Autodesk Fusion 360 part; units mm, degrees
(part 11 of 20)
  spline S1104 degree 3 poles (20.0046, -835.3457) (19.913, -835.5599) (19.6837, -836.0959) (19.6861, -836.6821) (19.6875, -837.034) knots 0 0 0 0 0.069271 0.173342 0.173342 0.173342 0.173342
sketch "Boceto14" plane through (0, -1, 0) normal (0, -1, 0) x (1, 0, 0)
  line L0 (28.545, -839.4996) -> (28.5449, -835.8775)
  line L1 (28.5449, -835.8775) -> (29.094, -835.8775)
  line L2 (29.094, -835.8775) -> (29.094, -836.3857)
  spline S0 degree 3 poles (29.094, -836.3857) (29.1559, -836.3011) (29.2808, -836.1306) (29.4582, -836.0156) (29.5476, -835.9576) knots 0 0 0 0 0.031158 0.062835 0.062835 0.062835 0.062835
  spline S1 degree 3 poles (29.5476, -835.9576) (29.6468, -835.9104) (29.8507, -835.8133) (30.0763, -835.8016) (30.1922, -835.7956) knots 0 0 0 0 0.032617 0.067048 0.067048 0.067048 0.067048
  spline S2 degree 3 poles (30.1922, -835.7956) (30.3167, -835.8003) (30.5491, -835.8092) (30.7561, -835.914) (30.8522, -835.9627) knots 0 0 0 0 0.036859 0.068796 0.068796 0.068796 0.068796
  spline S3 degree 3 poles (30.8522, -835.9627) (30.9319, -836.0244) (31.0928, -836.1491) (31.1743, -836.3357) (31.2154, -836.4299) knots 0 0 0 0 0.029725 0.060035 0.060035 0.060035 0.060035
  spline S4 degree 3 poles (31.2154, -836.4299) (31.3656, -836.245) (31.6567, -835.8864) (32.1131, -835.8252) (32.3341, -835.7955) knots 0 0 0 0 0.068625 0.133024 0.133024 0.133024 0.133024
  spline S5 degree 3 poles (32.3341, -835.7955) (32.4992, -835.8039) (32.8071, -835.8196) (33.0502, -836.007) (33.1629, -836.0939) knots 0 0 0 0 0.048244 0.08997 0.08997 0.08997 0.08997
  spline S6 degree 3 poles (33.1629, -836.0939) (33.2472, -836.2162) (33.4366, -836.4911) (33.4471, -836.8268) (33.4528, -837.0131) knots 0 0 0 0 0.043695 0.098195 0.098195 0.098195 0.098195
  line L3 (33.4528, -837.0131) -> (33.4529, -839.4994)
  line L4 (33.4529, -839.4994) -> (32.8424, -839.4995)
  line L5 (32.8424, -839.4995) -> (32.8423, -837.2177)
  spline S7 degree 3 poles (32.8423, -837.2177) (32.8423, -837.1115) (32.8423, -836.9322) (32.7999, -836.7583) (32.7826, -836.6874) knots 0 0 0 0 0.031711 0.053535 0.053535 0.053535 0.053535
  spline S8 degree 3 poles (32.7826, -836.6874) (32.7582, -836.6357) (32.7084, -836.5303) (32.6141, -836.4615) (32.5661, -836.4265) knots 0 0 0 0 0.016863 0.034394 0.034394 0.034394 0.034394
  spline S9 degree 3 poles (32.5661, -836.4265) (32.5103, -836.3976) (32.3949, -836.3379) (32.2649, -836.3311) (32.1977, -836.3276) knots 0 0 0 0 0.018597 0.038532 0.038532 0.038532 0.038532
  spline S10 degree 3 poles (32.1977, -836.3276) (32.0766, -836.3374) (31.8386, -836.3566) (31.654, -836.5076) (31.5633, -836.5817) knots 0 0 0 0 0.035532 0.069798 0.069798 0.069798 0.069798
  spline S11 degree 3 poles (31.5633, -836.5817) (31.49, -836.6884) (31.3229, -836.9316) (31.3153, -837.2285) (31.311, -837.3951) knots 0 0 0 0 0.038079 0.086792 0.086792 0.086792 0.086792
  line L6 (31.311, -837.3951) -> (31.311, -839.4995)
  line L7 (31.311, -839.4995) -> (30.6971, -839.4995)
  line L8 (30.6971, -839.4995) -> (30.697, -837.1462)
  spline S12 degree 3 poles (30.697, -837.1462) (30.6946, -837.0241) (30.6903, -836.8074) (30.5906, -836.6159) (30.547, -836.5323) knots 0 0 0 0 0.036008 0.063954 0.063954 0.063954 0.063954
  spline S13 degree 3 poles (30.547, -836.5323) (30.4847, -836.4727) (30.3485, -836.3423) (30.1589, -836.3328) (30.0558, -836.3277) knots 0 0 0 0 0.025037 0.054812 0.054812 0.054812 0.054812
  spline S14 degree 3 poles (30.0558, -836.3277) (29.9711, -836.3333) (29.8016, -836.3447) (29.6516, -836.4243) (29.5766, -836.4641) knots 0 0 0 0 0.025172 0.050327 0.050327 0.050327 0.050327
  spline S15 degree 3 poles (29.5766, -836.4641) (29.508, -836.5158) (29.3677, -836.6214) (29.2949, -836.7814) (29.2577, -836.8631) knots 0 0 0 0 0.025339 0.051812 0.051812 0.051812 0.051812
  spline S16 degree 3 poles (29.2577, -836.8631) (29.229, -836.9694) (29.1622, -837.217) (29.1601, -837.4738) (29.1589, -837.6203) knots 0 0 0 0 0.032907 0.076633 0.076633 0.076633 0.076633
  line L9 (29.1589, -837.6203) -> (29.1589, -839.4996)
  line L10 (29.1589, -839.4996) -> (28.545, -839.4996)
  line L11 (19.0617, -788.1561) -> (19.7063, -788.1015)
  spline S17 degree 3 poles (19.7063, -788.1015) (19.734, -788.2447) (19.7853, -788.5096) (19.9591, -788.7149) (20.0389, -788.8091) knots 0 0 0 0 0.042908 0.079365 0.079365 0.079365 0.079365
  spline S18 degree 3 poles (20.0389, -788.8091) (20.1311, -788.8783) (20.3177, -789.0182) (20.5504, -789.0368) (20.6682, -789.0461) knots 0 0 0 0 0.033826 0.068485 0.068485 0.068485 0.068485
  spline S19 degree 3 poles (20.6682, -789.0461) (20.8106, -789.0318) (21.0974, -789.003) (21.311, -788.8093) (21.4185, -788.7118) knots 0 0 0 0 0.041772 0.0841 0.0841 0.0841 0.0841
  spline S20 degree 3 poles (21.4185, -788.7118) (21.508, -788.5868) (21.6971, -788.3223) (21.7156, -787.9967) (21.7254, -787.825) knots 0 0 0 0 0.045186 0.095569 0.095569 0.095569 0.095569
  spline S21 degree 3 poles (21.7254, -787.825) (21.7163, -787.6627) (21.6992, -787.3564) (21.5163, -787.1114) (21.4303, -786.9963) knots 0 0 0 0 0.047557 0.089725 0.089725 0.089725 0.089725
  spline S22 degree 3 poles (21.4303, -786.9963) (21.3218, -786.9078) (21.0972, -786.7246) (20.8075, -786.7036) (20.6578, -786.6928) knots 0 0 0 0 0.040971 0.08482 0.08482 0.08482 0.08482
  spline S23 degree 3 poles (20.6578, -786.6928) (20.5622, -786.6979) (20.3748, -786.708) (20.2053, -786.7883) (20.1223, -786.8275) knots 0 0 0 0 0.028423 0.055689 0.055689 0.055689 0.055689
  spline S24 degree 3 poles (20.1223, -786.8275) (20.0475, -786.8751) (19.9006, -786.9683) (19.7977, -787.1085) (19.7472, -787.1772) knots 0 0 0 0 0.026342 0.051681 0.051681 0.051681 0.051681
  line L12 (19.7472, -787.1772) -> (19.1708, -787.1022)
  line L13 (19.1708, -787.1022) -> (19.6549, -784.5339)
  line L14 (19.6549, -784.5339) -> (22.1413, -784.5337)
  line L15 (22.1413, -784.5337) -> (22.1413, -785.1204)
  line L16 (22.1413, -785.1204) -> (20.1461, -785.1205)
  line L17 (20.1461, -785.1205) -> (19.8767, -786.4643)
  spline S25 degree 3 poles (19.8767, -786.4643) (20.0262, -786.3728) (20.3171, -786.1948) (20.6565, -786.165) (20.8215, -786.1505) knots 0 0 0 0 0.051785 0.100763 0.100763 0.100763 0.100763
  spline S26 degree 3 poles (20.8215, -786.1505) (21.0307, -786.1688) (21.4463, -786.2053) (21.7672, -786.4717) (21.9265, -786.604) knots 0 0 0 0 0.061424 0.122014 0.122014 0.122014 0.122014
  spline S27 degree 3 poles (21.9265, -786.604) (22.0578, -786.7694) (22.3287, -787.1108) (22.3605, -787.5461) (22.3768, -787.7704) knots 0 0 0 0 0.061868 0.127641 0.127641 0.127641 0.127641
  spline S28 degree 3 poles (22.3768, -787.7704) (22.3616, -787.9874) (22.3318, -788.4132) (22.0967, -788.7691) (21.9813, -788.9437) knots 0 0 0 0 0.064036 0.125703 0.125703 0.125703 0.125703
  spline S29 degree 3 poles (21.9813, -788.9437) (21.8036, -789.1208) (21.4405, -789.4825) (20.9292, -789.5278) (20.6682, -789.5509) knots 0 0 0 0 0.072854 0.148822 0.148822 0.148822 0.148822
  spline S30 degree 3 poles (20.6682, -789.5509) (20.455, -789.5382) (20.0475, -789.5138) (19.7138, -789.2803) (19.5546, -789.169) knots 0 0 0 0 0.062678 0.119794 0.119794 0.119794 0.119794
  spline S31 degree 3 poles (19.5546, -789.169) (19.426, -789.0286) (19.1617, -788.7403) (19.0956, -788.3542) (19.0617, -788.1561) knots 0 0 0 0 0.055877 0.114795 0.114795 0.114795 0.114795
  line L18 (27.4212, -788.1384) -> (28.0249, -788.2168)
  spline S32 degree 3 poles (28.0249, -788.2168) (27.9822, -788.4107) (27.9005, -788.7824) (27.6421, -789.0608) (27.5185, -789.194) knots 0 0 0 0 0.058356 0.111856 0.111856 0.111856 0.111856
  spline S33 degree 3 poles (27.5185, -789.194) (27.3724, -789.2969) (27.0723, -789.5084) (26.7057, -789.5339) (26.5175, -789.5471) knots 0 0 0 0 0.052559 0.107965 0.107965 0.107965 0.107965
  spline S34 degree 3 poles (26.5175, -789.5471) (26.2844, -789.5296) (25.8328, -789.4957) (25.4886, -789.2028) (25.322, -789.0611) knots 0 0 0 0 0.068154 0.132052 0.132052 0.132052 0.132052
  spline S35 degree 3 poles (25.322, -789.0611) (25.1905, -788.8704) (24.9026, -788.453) (24.8815, -787.9442) (24.87, -787.6679) knots 0 0 0 0 0.068157 0.149141 0.149141 0.149141 0.149141
  spline S36 degree 3 poles (24.87, -787.6679) (24.8763, -787.4827) (24.8883, -787.1302) (25.0077, -786.7986) (25.0643, -786.6413) knots 0 0 0 0 0.055211 0.105055 0.105055 0.105055 0.105055
  spline S37 degree 3 poles (25.0643, -786.6413) (25.1365, -786.5044) (25.2787, -786.2348) (25.5316, -786.0649) (25.656, -785.9813) knots 0 0 0 0 0.04564 0.089884 0.089884 0.089884 0.089884
  spline S38 degree 3 poles (25.656, -785.9813) (25.792, -785.9171) (26.0658, -785.7878) (26.3683, -785.7701) (26.5206, -785.7612) knots 0 0 0 0 0.044643 0.089955 0.089955 0.089955 0.089955
  spline S39 degree 3 poles (26.5206, -785.7612) (26.7043, -785.7706) (27.0522, -785.7884) (27.3468, -785.9726) (27.4858, -786.0596) knots 0 0 0 0 0.054149 0.102527 0.102527 0.102527 0.102527
  spline S40 degree 3 poles (27.4858, -786.0596) (27.6003, -786.1731) (27.8394, -786.4101) (27.9232, -786.7368) (27.9668, -786.9071) knots 0 0 0 0 0.047449 0.099081 0.099081 0.099081 0.099081
  line L19 (27.9668, -786.9071) -> (27.3699, -786.9992)
  spline S41 degree 3 poles (27.3699, -786.9992) (27.3391, -786.8878) (27.2816, -786.6804) (27.1356, -786.523) (27.0681, -786.4501) knots 0 0 0 0 0.034086 0.063475 0.063475 0.063475 0.063475
  spline S42 degree 3 poles (27.0681, -786.4501) (26.9911, -786.3964) (26.8338, -786.2867) (26.6423, -786.273) (26.5445, -786.266) knots 0 0 0 0 0.027619 0.056426 0.056426 0.056426 0.056426
  spline S43 degree 3 poles (26.5445, -786.266) (26.3979, -786.2791) (26.1087, -786.3048) (25.8958, -786.5016) (25.7908, -786.5986) knots 0 0 0 0 0.04285 0.084486 0.084486 0.084486 0.084486
  spline S44 degree 3 poles (25.7908, -786.5986) (25.7066, -786.7382) (25.5128, -787.0597) (25.5052, -787.4372) (25.501, -787.6508) knots 0 0 0 0 0.048123 0.11083 0.11083 0.11083 0.11083
  spline S45 degree 3 poles (25.501, -787.6508) (25.5046, -787.8666) (25.5109, -788.2453) (25.6995, -788.5712) (25.7807, -788.7115) knots 0 0 0 0 0.063398 0.111295 0.111295 0.111295 0.111295
  spline S46 degree 3 poles (25.7807, -788.7115) (25.8819, -788.808) (26.0864, -789.0031) (26.3682, -789.0291) (26.5106, -789.0423) knots 0 0 0 0 0.040675 0.082263 0.082263 0.082263 0.082263
  spline S47 degree 3 poles (26.5106, -789.0423) (26.625, -789.0341) (26.8478, -789.018) (27.0271, -788.8852) (27.1143, -788.8205) knots 0 0 0 0 0.033628 0.065508 0.065508 0.065508 0.065508
  spline S48 degree 3 poles (27.1143, -788.8205) (27.1883, -788.7306) (27.3518, -788.5319) (27.3967, -788.2775) (27.4212, -788.1384) knots 0 0 0 0 0.034396 0.07593 0.07593 0.07593 0.07593
  spline S49 degree 3 poles (21.7321, -737.034) (21.7357, -736.7657) (21.7422, -736.2825) (21.8615, -735.8147) (21.9145, -735.6066) knots 0 0 0 0 0.080152 0.144341 0.144341 0.144341 0.144341
  spline S50 degree 3 poles (21.9145, -735.6066) (21.9791, -735.4398) (22.1017, -735.1233) (22.3428, -734.8853) (22.4568, -734.7727) knots 0 0 0 0 0.052977 0.10048 0.10048 0.10048 0.10048
  spline S51 degree 3 poles (22.4568, -734.7727) (22.5882, -734.6872) (22.863, -734.5083) (23.1911, -734.4893) (23.3623, -734.4794) knots 0 0 0 0 0.046203 0.096661 0.096661 0.096661 0.096661
  spline S52 degree 3 poles (23.3623, -734.4794) (23.4901, -734.485) (23.7356, -734.4957) (23.9605, -734.5941) (24.0683, -734.6414) knots 0 0 0 0 0.037989 0.072993 0.072993 0.072993 0.072993
  spline S53 degree 3 poles (24.0683, -734.6414) (24.1655, -734.7021) (24.3629, -734.8252) (24.5001, -735.0132) (24.5697, -735.1086) knots 0 0 0 0 0.034048 0.069103 0.069103 0.069103 0.069103
  spline S54 degree 3 poles (24.5697, -735.1086) (24.633, -735.2196) (24.767, -735.4545) (24.841, -735.7148) (24.8801, -735.8521) knots 0 0 0 0 0.038176 0.080832 0.080832 0.080832 0.080832
  spline S55 degree 3 poles (24.8801, -735.8521) (24.9128, -736.0232) (24.9874, -736.4133) (24.9907, -736.8107) (24.9926, -737.0339) knots 0 0 0 0 0.052146 0.118926 0.118926 0.118926 0.118926
  spline S56 degree 3 poles (24.9926, -737.0339) (24.989, -737.3005) (24.9824, -737.7813) (24.8645, -738.247) (24.8119, -738.4544) knots 0 0 0 0 0.079639 0.143634 0.143634 0.143634 0.143634
  spline S57 degree 3 poles (24.8119, -738.4544) (24.7477, -738.6214) (24.6259, -738.9384) (24.3852, -739.1771) (24.2713, -739.2901) knots 0 0 0 0 0.052961 0.100531 0.100531 0.100531 0.100531
  spline S58 degree 3 poles (24.2713, -739.2901) (24.1397, -739.3761) (23.864, -739.5562) (23.5346, -739.5752) (23.3624, -739.5851) knots 0 0 0 0 0.046339 0.097057 0.097057 0.097057 0.097057
  spline S59 degree 3 poles (23.3624, -739.5851) (23.1362, -739.5658) (22.6949, -739.5281) (22.3801, -739.2179) (22.2267, -739.0667) knots 0 0 0 0 0.065835 0.128409 0.128409 0.128409 0.128409
  spline S60 degree 3 poles (22.2267, -739.0667) (22.0832, -738.7986) (21.7456, -738.1676) (21.737, -737.4479) (21.7321, -737.034) knots 0 0 0 0 0.090022 0.211899 0.211899 0.211899 0.211899
  line L20 (28.1509, -738.173) -> (28.7546, -738.2514)
  spline S61 degree 3 poles (28.7546, -738.2514) (28.7119, -738.4453) (28.6302, -738.8171) (28.3717, -739.0954) (28.2481, -739.2286) knots 0 0 0 0 0.058356 0.111856 0.111856 0.111856 0.111856
  spline S62 degree 3 poles (28.2481, -739.2286) (28.1021, -739.3315) (27.802, -739.543) (27.4353, -739.5685) (27.2471, -739.5816) knots 0 0 0 0 0.052559 0.107965 0.107965 0.107965 0.107965
  spline S63 degree 3 poles (27.2471, -739.5816) (27.0141, -739.5641) (26.5625, -739.5302) (26.2182, -739.2373) (26.0517, -739.0956) knots 0 0 0 0 0.068154 0.132052 0.132052 0.132052 0.132052
  spline S64 degree 3 poles (26.0517, -739.0956) (25.9201, -738.9049) (25.6323, -738.4875) (25.6112, -737.9787) (25.5997, -737.7024) knots 0 0 0 0 0.068157 0.149141 0.149141 0.149141 0.149141
  spline S65 degree 3 poles (25.5997, -737.7024) (25.6061, -737.5171) (25.6181, -737.1646) (25.7375, -736.8331) (25.7941, -736.6758) knots 0 0 0 0 0.055211 0.105055 0.105055 0.105055 0.105055
  spline S66 degree 3 poles (25.7941, -736.6758) (25.8663, -736.5389) (26.0085, -736.2693) (26.2614, -736.0994) (26.3859, -736.0158) knots 0 0 0 0 0.04564 0.089884 0.089884 0.089884 0.089884
  spline S67 degree 3 poles (26.3859, -736.0158) (26.5218, -735.9516) (26.7957, -735.8223) (27.0981, -735.8047) (27.2505, -735.7958) knots 0 0 0 0 0.044643 0.089956 0.089956 0.089956 0.089956
  spline S68 degree 3 poles (27.2505, -735.7958) (27.4342, -735.8052) (27.7821, -735.8229) (28.0767, -736.0072) (28.2157, -736.0942) knots 0 0 0 0 0.054149 0.102527 0.102527 0.102527 0.102527
  spline S69 degree 3 poles (28.2157, -736.0942) (28.3301, -736.2077) (28.5692, -736.4447) (28.6529, -736.7715) (28.6966, -736.9417) knots 0 0 0 0 0.047449 0.099081 0.099081 0.099081 0.099081
  line L21 (28.6966, -736.9417) -> (28.0997, -737.0338)
  spline S70 degree 3 poles (28.0997, -737.0338) (28.0689, -736.9224) (28.0114, -736.715) (27.8654, -736.5576) (27.7979, -736.4847) knots 0 0 0 0 0.034086 0.063475 0.063475 0.063475 0.063475
  spline S71 degree 3 poles (27.7979, -736.4847) (27.7209, -736.431) (27.5636, -736.3213) (27.3721, -736.3076) (27.2743, -736.3006) knots 0 0 0 0 0.027619 0.056426 0.056426 0.056426 0.056426
  spline S72 degree 3 poles (27.2743, -736.3006) (27.1277, -736.3136) (26.8385, -736.3393) (26.6256, -736.5361) (26.5206, -736.6331) knots 0 0 0 0 0.04285 0.084486 0.084486 0.084486 0.084486
  spline S73 degree 3 poles (26.5206, -736.6331) (26.4364, -736.7727) (26.2425, -737.0942) (26.235, -737.4717) (26.2307, -737.6853) knots 0 0 0 0 0.048123 0.11083 0.11083 0.11083 0.11083
  spline S74 degree 3 poles (26.2307, -737.6853) (26.2343, -737.9011) (26.2406, -738.2798) (26.4292, -738.6057) (26.5104, -738.746) knots 0 0 0 0 0.063398 0.111295 0.111295 0.111295 0.111295
  spline S75 degree 3 poles (26.5104, -738.746) (26.6116, -738.8425) (26.8161, -739.0376) (27.0979, -739.0637) (27.2403, -739.0768) knots 0 0 0 0 0.040675 0.082263 0.082263 0.082263 0.082263
  spline S76 degree 3 poles (27.2403, -739.0768) (27.3547, -739.0686) (27.5775, -739.0526) (27.7568, -738.9198) (27.844, -738.8551) knots 0 0 0 0 0.033628 0.065508 0.065508 0.065508 0.065508
  spline S77 degree 3 poles (27.844, -738.8551) (27.918, -738.7651) (28.0815, -738.5665) (28.1264, -738.3121) (28.1509, -738.173) knots 0 0 0 0 0.034396 0.07593 0.07593 0.07593 0.07593
  line L22 (21.7306, -688.1902) -> (22.3752, -688.1357)
  spline S78 degree 3 poles (22.3752, -688.1357) (22.4029, -688.2789) (22.4541, -688.5438) (22.6279, -688.7491) (22.7077, -688.8434) knots 0 0 0 0 0.042908 0.079365 0.079365 0.079365 0.079365
  spline S79 degree 3 poles (22.7077, -688.8434) (22.7999, -688.9125) (22.9865, -689.0525) (23.2192, -689.071) (23.337, -689.0804) knots 0 0 0 0 0.033826 0.068485 0.068485 0.068485 0.068485
  spline S80 degree 3 poles (23.337, -689.0804) (23.4794, -689.0661) (23.7662, -689.0373) (23.9798, -688.8436) (24.0873, -688.7462) knots 0 0 0 0 0.041772 0.0841 0.0841 0.0841 0.0841
  spline S81 degree 3 poles (24.0873, -688.7462) (24.1768, -688.6211) (24.366, -688.3566) (24.3845, -688.031) (24.3943, -687.8594) knots 0 0 0 0 0.045186 0.095569 0.095569 0.095569 0.095569
  spline S82 degree 3 poles (24.3943, -687.8594) (24.3852, -687.697) (24.3681, -687.3907) (24.1852, -687.1457) (24.0992, -687.0306) knots 0 0 0 0 0.047557 0.089725 0.089725 0.089725 0.089725
  spline S83 degree 3 poles (24.0992, -687.0306) (23.9907, -686.9421) (23.7662, -686.7589) (23.4765, -686.7379) (23.3267, -686.7271) knots 0 0 0 0 0.040971 0.08482 0.08482 0.08482 0.08482
  spline S84 degree 3 poles (23.3267, -686.7271) (23.2311, -686.7322) (23.0437, -686.7423) (22.8742, -686.8225) (22.7912, -686.8618) knots 0 0 0 0 0.028423 0.055689 0.055689 0.055689 0.055689
  spline S85 degree 3 poles (22.7912, -686.8618) (22.7164, -686.9093) (22.5695, -687.0026) (22.4666, -687.1427) (22.4161, -687.2114) knots 0 0 0 0 0.026342 0.051681 0.051681 0.051681 0.051681
  line L23 (22.4161, -687.2114) -> (21.8397, -687.1364)
  line L24 (21.8397, -687.1364) -> (22.324, -684.5681)
  line L25 (22.324, -684.5681) -> (24.8103, -684.5681)
  line L26 (24.8103, -684.5681) -> (24.8103, -685.1547)
  line L27 (24.8103, -685.1547) -> (22.8151, -685.1548)
  line L28 (22.8151, -685.1548) -> (22.5457, -686.4986)
  spline S86 degree 3 poles (22.5457, -686.4986) (22.6952, -686.4071) (22.986, -686.229) (23.3254, -686.1992) (23.4904, -686.1848) knots 0 0 0 0 0.051785 0.100763 0.100763 0.100763 0.100763
  spline S87 degree 3 poles (23.4904, -686.1848) (23.6997, -686.2031) (24.1153, -686.2396) (24.4361, -686.5061) (24.5955, -686.6384) knots 0 0 0 0 0.061424 0.122014 0.122014 0.122014 0.122014
  spline S88 degree 3 poles (24.5955, -686.6384) (24.7267, -686.8038) (24.9976, -687.1451) (25.0293, -687.5805) (25.0457, -687.8048) knots 0 0 0 0 0.061868 0.127641 0.127641 0.127641 0.127641
  spline S89 degree 3 poles (25.0457, -687.8048) (25.0305, -688.0218) (25.0006, -688.4476) (24.7654, -688.8035) (24.6501, -688.9781) knots 0 0 0 0 0.064036 0.125703 0.125703 0.125703 0.125703
  spline S90 degree 3 poles (24.6501, -688.9781) (24.4723, -689.1551) (24.1093, -689.5168) (23.598, -689.5621) (23.337, -689.5852) knots 0 0 0 0 0.072854 0.148822 0.148822 0.148822 0.148822
  spline S91 degree 3 poles (23.337, -689.5852) (23.1238, -689.5724) (22.7162, -689.5481) (22.3825, -689.3145) (22.2234, -689.2032) knots 0 0 0 0 0.062678 0.119794 0.119794 0.119794 0.119794
  spline S92 degree 3 poles (22.2234, -689.2032) (22.0948, -689.0628) (21.8305, -688.7745) (21.7644, -688.3884) (21.7306, -688.1902) knots 0 0 0 0 0.055877 0.114795 0.114795 0.114795 0.114795
  line L29 (28.1494, -688.1731) -> (28.7531, -688.2516)
  spline S93 degree 3 poles (28.7531, -688.2516) (28.7104, -688.4455) (28.6286, -688.8172) (28.3702, -689.0956) (28.2466, -689.2287) knots 0 0 0 0 0.058356 0.111856 0.111856 0.111856 0.111856
  spline S94 degree 3 poles (28.2466, -689.2287) (28.1005, -689.3317) (27.8004, -689.5431) (27.4337, -689.5686) (27.2456, -689.5817) knots 0 0 0 0 0.052559 0.107965 0.107965 0.107965 0.107965
  spline S95 degree 3 poles (27.2456, -689.5817) (27.0125, -689.5642) (26.5609, -689.5303) (26.2167, -689.2374) (26.0501, -689.0957) knots 0 0 0 0 0.068154 0.132052 0.132052 0.132052 0.132052
  spline S96 degree 3 poles (26.0501, -689.0957) (25.9186, -688.905) (25.6307, -688.4876) (25.6097, -687.9788) (25.5982, -687.7025) knots 0 0 0 0 0.068157 0.149141 0.149141 0.149141 0.149141
  spline S97 degree 3 poles (25.5982, -687.7025) (25.6045, -687.5172) (25.6165, -687.1647) (25.7359, -686.8332) (25.7926, -686.6759) knots 0 0 0 0 0.055211 0.105055 0.105055 0.105055 0.105055
  spline S98 degree 3 poles (25.7926, -686.6759) (25.8648, -686.539) (26.007, -686.2694) (26.2599, -686.0995) (26.3843, -686.0159) knots 0 0 0 0 0.04564 0.089884 0.089884 0.089884 0.089884
  spline S99 degree 3 poles (26.3843, -686.0159) (26.5203, -685.9517) (26.7942, -685.8225) (27.0966, -685.8048) (27.2489, -685.7959) knots 0 0 0 0 0.044643 0.089955 0.089955 0.089955 0.089955
  spline S100 degree 3 poles (27.2489, -685.7959) (27.4327, -685.8053) (27.7805, -685.8231) (28.0751, -686.0074) (28.2142, -686.0943) knots 0 0 0 0 0.054149 0.102527 0.102527 0.102527 0.102527
  spline S101 degree 3 poles (28.2142, -686.0943) (28.3286, -686.2078) (28.5677, -686.4449) (28.6514, -686.7716) (28.6951, -686.9419) knots 0 0 0 0 0.047449 0.099081 0.099081 0.099081 0.099081
  line L30 (28.6951, -686.9419) -> (28.0982, -687.034)
  spline S102 degree 3 poles (28.0982, -687.034) (28.0673, -686.9226) (28.0099, -686.7151) (27.8639, -686.5577) (27.7964, -686.4849) knots 0 0 0 0 0.034086 0.063475 0.063475 0.063475 0.063475
  spline S103 degree 3 poles (27.7964, -686.4849) (27.7194, -686.4311) (27.5621, -686.3214) (27.3706, -686.3077) (27.2728, -686.3007) knots 0 0 0 0 0.027619 0.056426 0.056426 0.056426 0.056426
  spline S104 degree 3 poles (27.2728, -686.3007) (27.1262, -686.3137) (26.837, -686.3394) (26.624, -686.5362) (26.5191, -686.6332) knots 0 0 0 0 0.04285 0.084486 0.084486 0.084486 0.084486
  spline S105 degree 3 poles (26.5191, -686.6332) (26.4349, -686.7728) (26.241, -687.0943) (26.2335, -687.4718) (26.2292, -687.6854) knots 0 0 0 0 0.048123 0.11083 0.11083 0.11083 0.11083
  spline S106 degree 3 poles (26.2292, -687.6854) (26.2328, -687.9012) (26.2391, -688.2799) (26.4277, -688.6059) (26.5089, -688.7461) knots 0 0 0 0 0.063398 0.111295 0.111295 0.111295 0.111295
  spline S107 degree 3 poles (26.5089, -688.7461) (26.61, -688.8426) (26.8146, -689.0378) (27.0963, -689.0638) (27.2387, -689.0769) knots 0 0 0 0 0.040675 0.082263 0.082263 0.082263 0.082263
  spline S108 degree 3 poles (27.2387, -689.0769) (27.3531, -689.0687) (27.576, -689.0527) (27.7552, -688.9199) (27.8424, -688.8553) knots 0 0 0 0 0.033628 0.065508 0.065508 0.065508 0.065508
  spline S109 degree 3 poles (27.8424, -688.8553) (27.9165, -688.7653) (28.0799, -688.5666) (28.1248, -688.3123) (28.1494, -688.1731) knots 0 0 0 0 0.034396 0.07593 0.07593 0.07593 0.07593
  spline S110 degree 3 poles (22.0101, -637.034) (22.0137, -636.7656) (22.0202, -636.2824) (22.1394, -635.8146) (22.1925, -635.6066) knots 0 0 0 0 0.080152 0.144341 0.144341 0.144341 0.144341
  spline S111 degree 3 poles (22.1925, -635.6066) (22.2571, -635.4397) (22.3796, -635.1233) (22.6208, -634.8852) (22.7348, -634.7727) knots 0 0 0 0 0.052977 0.10048 0.10048 0.10048 0.10048
  spline S112 degree 3 poles (22.7348, -634.7727) (22.8661, -634.6872) (23.141, -634.5083) (23.469, -634.4893) (23.6403, -634.4794) knots 0 0 0 0 0.046203 0.096661 0.096661 0.096661 0.096661
  spline S113 degree 3 poles (23.6403, -634.4794) (23.7681, -634.4849) (24.0136, -634.4956) (24.2384, -634.5941) (24.3463, -634.6413) knots 0 0 0 0 0.037989 0.072993 0.072993 0.072993 0.072993
  spline S114 degree 3 poles (24.3463, -634.6413) (24.4435, -634.702) (24.6409, -634.8252) (24.7781, -635.0132) (24.8477, -635.1086) knots 0 0 0 0 0.034048 0.069103 0.069103 0.069103 0.069103
  spline S115 degree 3 poles (24.8477, -635.1086) (24.911, -635.2195) (25.045, -635.4544) (25.119, -635.7147) (25.1581, -635.8521) knots 0 0 0 0 0.038176 0.080832 0.080832 0.080832 0.080832
  spline S116 degree 3 poles (25.1581, -635.8521) (25.1908, -636.0231) (25.2653, -636.4133) (25.2687, -636.8107) (25.2706, -637.0339) knots 0 0 0 0 0.052146 0.118926 0.118926 0.118926 0.118926
  spline S117 degree 3 poles (25.2706, -637.0339) (25.267, -637.3005) (25.2604, -637.7813) (25.1425, -638.2469) (25.0899, -638.4544) knots 0 0 0 0 0.079639 0.143634 0.143634 0.143634 0.143634
  spline S118 degree 3 poles (25.0899, -638.4544) (25.0257, -638.6214) (24.9039, -638.9383) (24.6632, -639.1771) (24.5493, -639.29) knots 0 0 0 0 0.052961 0.100531 0.100531 0.100531 0.100531
  spline S119 degree 3 poles (24.5493, -639.29) (24.4177, -639.376) (24.142, -639.5562) (23.8126, -639.5752) (23.6404, -639.5851) knots 0 0 0 0 0.046339 0.097057 0.097057 0.097057 0.097057
  spline S120 degree 3 poles (23.6404, -639.5851) (23.4142, -639.5658) (22.9729, -639.5281) (22.6581, -639.2179) (22.5047, -639.0667) knots 0 0 0 0 0.065835 0.128409 0.128409 0.128409 0.128409
  spline S121 degree 3 poles (22.5047, -639.0667) (22.3612, -638.7986) (22.0236, -638.1676) (22.015, -637.4479) (22.0101, -637.034) knots 0 0 0 0 0.090022 0.211899 0.211899 0.211899 0.211899
  line L31 (28.4289, -638.1729) -> (29.0326, -638.2514)
  spline S122 degree 3 poles (29.0326, -638.2514) (28.9899, -638.4453) (28.9082, -638.817) (28.6498, -639.0954) (28.5262, -639.2285) knots 0 0 0 0 0.058356 0.111856 0.111856 0.111856 0.111856
  spline S123 degree 3 poles (28.5262, -639.2285) (28.3801, -639.3315) (28.08, -639.5429) (27.7133, -639.5685) (27.5251, -639.5816) knots 0 0 0 0 0.052559 0.107965 0.107965 0.107965 0.107965
  spline S124 degree 3 poles (27.5251, -639.5816) (27.2921, -639.5641) (26.8405, -639.5301) (26.4963, -639.2373) (26.3297, -639.0956) knots 0 0 0 0 0.068154 0.132052 0.132052 0.132052 0.132052
  spline S125 degree 3 poles (26.3297, -639.0956) (26.1981, -638.9048) (25.9103, -638.4875) (25.8892, -637.9786) (25.8777, -637.7023) knots 0 0 0 0 0.068157 0.149141 0.149141 0.149141 0.149141
  spline S126 degree 3 poles (25.8777, -637.7023) (25.8841, -637.5171) (25.8961, -637.1646) (26.0155, -636.833) (26.0721, -636.6757) knots 0 0 0 0 0.055211 0.105055 0.105055 0.105055 0.105055
  spline S127 degree 3 poles (26.0721, -636.6757) (26.1443, -636.5388) (26.2865, -636.2692) (26.5394, -636.0994) (26.6639, -636.0158) knots 0 0 0 0 0.04564 0.089884 0.089884 0.089884 0.089884
  spline S128 degree 3 poles (26.6639, -636.0158) (26.7998, -635.9516) (27.0737, -635.8223) (27.3761, -635.8046) (27.5284, -635.7958) knots 0 0 0 0 0.044643 0.089955 0.089955 0.089955 0.089955
  spline S129 degree 3 poles (27.5284, -635.7958) (27.7122, -635.8051) (28.0601, -635.8229) (28.3547, -636.0072) (28.4937, -636.0942) knots 0 0 0 0 0.054149 0.102527 0.102527 0.102527 0.102527
  spline S130 degree 3 poles (28.4937, -636.0942) (28.6081, -636.2077) (28.8472, -636.4447) (28.9309, -636.7714) (28.9746, -636.9417) knots 0 0 0 0 0.047449 0.099081 0.099081 0.099081 0.099081
  line L32 (28.9746, -636.9417) -> (28.3777, -637.0338)
  spline S131 degree 3 poles (28.3777, -637.0338) (28.3469, -636.9224) (28.2894, -636.715) (28.1434, -636.5576) (28.0759, -636.4847) knots 0 0 0 0 0.034086 0.063475 0.063475 0.063475 0.063475
  spline S132 degree 3 poles (28.0759, -636.4847) (27.9989, -636.431) (27.8416, -636.3213) (27.6501, -636.3075) (27.5523, -636.3005) knots 0 0 0 0 0.027619 0.056426 0.056426 0.056426 0.056426
  spline S133 degree 3 poles (27.5523, -636.3005) (27.4057, -636.3136) (27.1165, -636.3393) (26.9036, -636.5361) (26.7986, -636.6331) knots 0 0 0 0 0.04285 0.084486 0.084486 0.084486 0.084486
  spline S134 degree 3 poles (26.7986, -636.6331) (26.7144, -636.7727) (26.5205, -637.0941) (26.513, -637.4717) (26.5087, -637.6853) knots 0 0 0 0 0.048123 0.11083 0.11083 0.11083 0.11083
  spline S135 degree 3 poles (26.5087, -637.6853) (26.5123, -637.901) (26.5186, -638.2798) (26.7072, -638.6057) (26.7884, -638.746) knots 0 0 0 0 0.063398 0.111295 0.111295 0.111295 0.111295
  spline S136 degree 3 poles (26.7884, -638.746) (26.8896, -638.8425) (27.0941, -639.0376) (27.3759, -639.0636) (27.5183, -639.0768) knots 0 0 0 0 0.040675 0.082263 0.082263 0.082263 0.082263
  spline S137 degree 3 poles (27.5183, -639.0768) (27.6327, -639.0686) (27.8555, -639.0526) (28.0348, -638.9197) (28.122, -638.8551) knots 0 0 0 0 0.033628 0.065508 0.065508 0.065508 0.065508
  spline S138 degree 3 poles (28.122, -638.8551) (28.196, -638.7651) (28.3595, -638.5665) (28.4044, -638.3121) (28.4289, -638.1729) knots 0 0 0 0 0.034396 0.07593 0.07593 0.07593 0.07593
  line L33 (22.0076, -588.1903) -> (22.6523, -588.1357)
  spline S139 degree 3 poles (22.6523, -588.1357) (22.68, -588.2789) (22.7312, -588.5439) (22.905, -588.7491) (22.9848, -588.8434) knots 0 0 0 0 0.042908 0.079365 0.079365 0.079365 0.079365
  spline S140 degree 3 poles (22.9848, -588.8434) (23.077, -588.9125) (23.2636, -589.0525) (23.4963, -589.0711) (23.6141, -589.0804) knots 0 0 0 0 0.033826 0.068485 0.068485 0.068485 0.068485
  spline S141 degree 3 poles (23.6141, -589.0804) (23.7565, -589.0662) (24.0433, -589.0374) (24.2569, -588.8437) (24.3644, -588.7462) knots 0 0 0 0 0.041772 0.0841 0.0841 0.0841 0.0841
  spline S142 degree 3 poles (24.3644, -588.7462) (24.4539, -588.6211) (24.6431, -588.3567) (24.6616, -588.0311) (24.6714, -587.8594) knots 0 0 0 0 0.045186 0.095569 0.095569 0.095569 0.095569
  spline S143 degree 3 poles (24.6714, -587.8594) (24.6623, -587.6971) (24.6452, -587.3908) (24.4623, -587.1458) (24.3763, -587.0306) knots 0 0 0 0 0.047557 0.089725 0.089725 0.089725 0.089725
  spline S144 degree 3 poles (24.3763, -587.0306) (24.2678, -586.9421) (24.0433, -586.7589) (23.7536, -586.7379) (23.6038, -586.7271) knots 0 0 0 0 0.040971 0.08482 0.08482 0.08482 0.08482
  spline S145 degree 3 poles (23.6038, -586.7271) (23.5082, -586.7322) (23.3208, -586.7423) (23.1513, -586.8225) (23.0683, -586.8618) knots 0 0 0 0 0.028423 0.055689 0.055689 0.055689 0.055689
  spline S146 degree 3 poles (23.0683, -586.8618) (22.9935, -586.9094) (22.8466, -587.0026) (22.7437, -587.1427) (22.6932, -587.2114) knots 0 0 0 0 0.026342 0.051681 0.051681 0.051681 0.051681
  line L34 (22.6932, -587.2114) -> (22.1168, -587.1364)
  line L35 (22.1168, -587.1364) -> (22.6011, -584.5682)
  line L36 (22.6011, -584.5682) -> (25.0874, -584.5682)
  line L37 (25.0874, -584.5682) -> (25.0874, -585.1548)
  line L38 (25.0874, -585.1548) -> (23.0922, -585.1548)
  line L39 (23.0922, -585.1548) -> (22.8228, -586.4986)
  spline S147 degree 3 poles (22.8228, -586.4986) (22.9723, -586.4071) (23.2631, -586.2291) (23.6026, -586.1993) (23.7675, -586.1848) knots 0 0 0 0 0.051785 0.100763 0.100763 0.100763 0.100763
  spline S148 degree 3 poles (23.7675, -586.1848) (23.9768, -586.2032) (24.3924, -586.2397) (24.7132, -586.5061) (24.8726, -586.6384) knots 0 0 0 0 0.061424 0.122014 0.122014 0.122014 0.122014
  spline S149 degree 3 poles (24.8726, -586.6384) (25.0039, -586.8039) (25.2747, -587.1452) (25.3064, -587.5805) (25.3228, -587.8049) knots 0 0 0 0 0.061868 0.12764 0.12764 0.12764 0.12764
  spline S150 degree 3 poles (25.3228, -587.8049) (25.3076, -588.0218) (25.2777, -588.4477) (25.0425, -588.8035) (24.9272, -588.9781) knots 0 0 0 0 0.064036 0.125703 0.125703 0.125703 0.125703
  spline S151 degree 3 poles (24.9272, -588.9781) (24.7494, -589.1552) (24.3864, -589.5168) (23.8751, -589.5621) (23.6141, -589.5852) knots 0 0 0 0 0.072854 0.148822 0.148822 0.148822 0.148822
  spline S152 degree 3 poles (23.6141, -589.5852) (23.4008, -589.5725) (22.9933, -589.5481) (22.6596, -589.3146) (22.5005, -589.2032) knots 0 0 0 0 0.062678 0.119794 0.119794 0.119794 0.119794
  spline S153 degree 3 poles (22.5005, -589.2032) (22.3719, -589.0629) (22.1076, -588.7745) (22.0415, -588.3884) (22.0076, -588.1903) knots 0 0 0 0 0.055877 0.114795 0.114795 0.114795 0.114795
  line L40 (28.4265, -588.1732) -> (29.0302, -588.2516)
  spline S154 degree 3 poles (29.0302, -588.2516) (28.9875, -588.4456) (28.9057, -588.8173) (28.6473, -589.0956) (28.5237, -589.2288) knots 0 0 0 0 0.058356 0.111856 0.111856 0.111856 0.111856
  spline S155 degree 3 poles (28.5237, -589.2288) (28.3776, -589.3317) (28.0775, -589.5432) (27.7108, -589.5687) (27.5227, -589.5818) knots 0 0 0 0 0.052559 0.107965 0.107965 0.107965 0.107965
  spline S156 degree 3 poles (27.5227, -589.5818) (27.2896, -589.5643) (26.838, -589.5304) (26.4938, -589.2375) (26.3272, -589.0958) knots 0 0 0 0 0.068154 0.132052 0.132052 0.132052 0.132052
  spline S157 degree 3 poles (26.3272, -589.0958) (26.1957, -588.905) (25.9078, -588.4877) (25.8867, -587.9788) (25.8753, -587.7025) knots 0 0 0 0 0.068157 0.149141 0.149141 0.149141 0.149141
  spline S158 degree 3 poles (25.8753, -587.7025) (25.8816, -587.5173) (25.8936, -587.1648) (26.013, -586.8332) (26.0697, -586.6759) knots 0 0 0 0 0.055211 0.105055 0.105055 0.105055 0.105055
  spline S159 degree 3 poles (26.0697, -586.6759) (26.1419, -586.539) (26.2841, -586.2694) (26.537, -586.0996) (26.6615, -586.016) knots 0 0 0 0 0.04564 0.089884 0.089884 0.089884 0.089884
  spline S160 degree 3 poles (26.6615, -586.016) (26.7974, -585.9518) (27.0713, -585.8225) (27.3737, -585.8049) (27.526, -585.796) knots 0 0 0 0 0.044643 0.089955 0.089955 0.089955 0.089955
  spline S161 degree 3 poles (27.526, -585.796) (27.7098, -585.8054) (28.0577, -585.8231) (28.3523, -586.0074) (28.4913, -586.0944) knots 0 0 0 0 0.054149 0.102527 0.102527 0.102527 0.102527
  spline S162 degree 3 poles (28.4913, -586.0944) (28.6057, -586.2079) (28.8448, -586.4449) (28.9285, -586.7717) (28.9722, -586.9419) knots 0 0 0 0 0.047449 0.099081 0.099081 0.099081 0.099081
  line L41 (28.9722, -586.9419) -> (28.3753, -587.034)
  spline S163 degree 3 poles (28.3753, -587.034) (28.3444, -586.9226) (28.287, -586.7152) (28.141, -586.5578) (28.0735, -586.4849) knots 0 0 0 0 0.034086 0.063475 0.063475 0.063475 0.063475
  spline S164 degree 3 poles (28.0735, -586.4849) (27.9965, -586.4312) (27.8392, -586.3215) (27.6477, -586.3078) (27.5499, -586.3008) knots 0 0 0 0 0.027619 0.056426 0.056426 0.056426 0.056426
  spline S165 degree 3 poles (27.5499, -586.3008) (27.4033, -586.3138) (27.1141, -586.3395) (26.9011, -586.5363) (26.7962, -586.6333) knots 0 0 0 0 0.04285 0.084486 0.084486 0.084486 0.084486
  spline S166 degree 3 poles (26.7962, -586.6333) (26.712, -586.7729) (26.5181, -587.0943) (26.5106, -587.4719) (26.5063, -587.6855) knots 0 0 0 0 0.048123 0.11083 0.11083 0.11083 0.11083
  spline S167 degree 3 poles (26.5063, -587.6855) (26.5099, -587.9012) (26.5162, -588.28) (26.7048, -588.6059) (26.786, -588.7462) knots 0 0 0 0 0.063398 0.111295 0.111295 0.111295 0.111295
  spline S168 degree 3 poles (26.786, -588.7462) (26.8871, -588.8427) (27.0917, -589.0378) (27.3734, -589.0639) (27.5158, -589.077) knots 0 0 0 0 0.040675 0.082263 0.082263 0.082263 0.082263
  spline S169 degree 3 poles (27.5158, -589.077) (27.6302, -589.0688) (27.8531, -589.0528) (28.0323, -588.92) (28.1195, -588.8553) knots 0 0 0 0 0.033628 0.065508 0.065508 0.065508 0.065508
  spline S170 degree 3 poles (28.1195, -588.8553) (28.1936, -588.7653) (28.357, -588.5667) (28.4019, -588.3123) (28.4265, -588.1732) knots 0 0 0 0 0.034396 0.07593 0.07593 0.07593 0.07593
  spline S171 degree 3 poles (21.9704, -537.0337) (21.974, -536.7654) (21.9805, -536.2822) (22.0997, -535.8144) (22.1528, -535.6063) knots 0 0 0 0 0.080152 0.144341 0.144341 0.144341 0.144341
  spline S172 degree 3 poles (22.1528, -535.6063) (22.2174, -535.4395) (22.3399, -535.123) (22.581, -534.8849) (22.695, -534.7724) knots 0 0 0 0 0.052977 0.10048 0.10048 0.10048 0.10048
  spline S173 degree 3 poles (22.695, -534.7724) (22.8264, -534.6869) (23.1012, -534.508) (23.4293, -534.4889) (23.6005, -534.479) knots 0 0 0 0 0.046203 0.096661 0.096661 0.096661 0.096661
  spline S174 degree 3 poles (23.6005, -534.479) (23.7283, -534.4846) (23.9738, -534.4953) (24.1987, -534.5937) (24.3065, -534.6409) knots 0 0 0 0 0.037989 0.072993 0.072993 0.072993 0.072993
  spline S175 degree 3 poles (24.3065, -534.6409) (24.4038, -534.7016) (24.6011, -534.8248) (24.7383, -535.0128) (24.8079, -535.1082) knots 0 0 0 0 0.034048 0.069103 0.069103 0.069103 0.069103
  spline S176 degree 3 poles (24.8079, -535.1082) (24.8712, -535.2191) (25.0053, -535.454) (25.0793, -535.7143) (25.1184, -535.8517) knots 0 0 0 0 0.038176 0.080832 0.080832 0.080832 0.080832
  spline S177 degree 3 poles (25.1184, -535.8517) (25.1511, -536.0227) (25.2257, -536.4128) (25.2291, -536.8103) (25.231, -537.0334) knots 0 0 0 0 0.052146 0.118926 0.118926 0.118926 0.118926
  spline S178 degree 3 poles (25.231, -537.0334) (25.2274, -537.3) (25.2208, -537.7808) (25.1029, -538.2465) (25.0504, -538.454) knots 0 0 0 0 0.079639 0.143634 0.143634 0.143634 0.143634
  spline S179 degree 3 poles (25.0504, -538.454) (24.9862, -538.6209) (24.8644, -538.9379) (24.6237, -539.1767) (24.5098, -539.2896) knots 0 0 0 0 0.052961 0.100531 0.100531 0.100531 0.100531
  spline S180 degree 3 poles (24.5098, -539.2896) (24.3782, -539.3756) (24.1025, -539.5558) (23.7731, -539.5748) (23.6009, -539.5847) knots 0 0 0 0 0.046339 0.097057 0.097057 0.097057 0.097057
  spline S181 degree 3 poles (23.6009, -539.5847) (23.3747, -539.5654) (22.9334, -539.5278) (22.6186, -539.2176) (22.4651, -539.0664) knots 0 0 0 0 0.065835 0.128409 0.128409 0.128409 0.128409
  spline S182 degree 3 poles (22.4651, -539.0664) (22.3217, -538.7983) (21.984, -538.1673) (21.9754, -537.4476) (21.9704, -537.0337) knots 0 0 0 0 0.090022 0.211899 0.211899 0.211899 0.211899
  line L42 (28.3894, -538.1723) -> (28.993, -538.2507)
  spline S183 degree 3 poles (28.993, -538.2507) (28.9504, -538.4446) (28.8686, -538.8163) (28.6102, -539.0947) (28.4866, -539.2279) knots 0 0 0 0 0.058356 0.111856 0.111856 0.111856 0.111856
  spline S184 degree 3 poles (28.4866, -539.2279) (28.3406, -539.3309) (28.0405, -539.5423) (27.6738, -539.5679) (27.4857, -539.581) knots 0 0 0 0 0.052559 0.107965 0.107965 0.107965 0.107965
  spline S185 degree 3 poles (27.4857, -539.581) (27.2526, -539.5635) (26.801, -539.5296) (26.4568, -539.2368) (26.2902, -539.0951) knots 0 0 0 0 0.068154 0.132052 0.132052 0.132052 0.132052
  spline S186 degree 3 poles (26.2902, -539.0951) (26.1586, -538.9043) (25.8707, -538.487) (25.8496, -537.9782) (25.8382, -537.7019) knots 0 0 0 0 0.068157 0.149141 0.149141 0.149141 0.149141
  spline S187 degree 3 poles (25.8382, -537.7019) (25.8445, -537.5166) (25.8564, -537.1641) (25.9758, -536.8326) (26.0325, -536.6752) knots 0 0 0 0 0.055211 0.105055 0.105055 0.105055 0.105055
  spline S188 degree 3 poles (26.0325, -536.6752) (26.1047, -536.5383) (26.2468, -536.2687) (26.4997, -536.0988) (26.6242, -536.0152) knots 0 0 0 0 0.04564 0.089884 0.089884 0.089884 0.089884
  spline S189 degree 3 poles (26.6242, -536.0152) (26.7601, -535.9511) (27.034, -535.8218) (27.3364, -535.8041) (27.4887, -535.7952) knots 0 0 0 0 0.044643 0.089956 0.089956 0.089956 0.089956
  spline S190 degree 3 poles (27.4887, -535.7952) (27.6725, -535.8045) (28.0203, -535.8223) (28.315, -536.0066) (28.454, -536.0935) knots 0 0 0 0 0.054149 0.102527 0.102527 0.102527 0.102527
  spline S191 degree 3 poles (28.454, -536.0935) (28.5685, -536.207) (28.8075, -536.444) (28.8913, -536.7708) (28.935, -536.941) knots 0 0 0 0 0.047449 0.099081 0.099081 0.099081 0.099081
  line L43 (28.935, -536.941) -> (28.3381, -537.0332)
  spline S192 degree 3 poles (28.3381, -537.0332) (28.3072, -536.9218) (28.2497, -536.7143) (28.1038, -536.557) (28.0362, -536.4841) knots 0 0 0 0 0.034086 0.063475 0.063475 0.063475 0.063475
  spline S193 degree 3 poles (28.0362, -536.4841) (27.9592, -536.4304) (27.8019, -536.3207) (27.6104, -536.3069) (27.5127, -536.2999) knots 0 0 0 0 0.027619 0.056426 0.056426 0.056426 0.056426
  spline S194 degree 3 poles (27.5127, -536.2999) (27.366, -536.313) (27.0769, -536.3387) (26.8639, -536.5356) (26.7589, -536.6325) knots 0 0 0 0 0.04285 0.084486 0.084486 0.084486 0.084486
  spline S195 degree 3 poles (26.7589, -536.6325) (26.6748, -536.7721) (26.4809, -537.0936) (26.4734, -537.4712) (26.4691, -537.6848) knots 0 0 0 0 0.048123 0.11083 0.11083 0.11083 0.11083
  spline S196 degree 3 poles (26.4691, -537.6848) (26.4727, -537.9005) (26.4791, -538.2793) (26.6677, -538.6052) (26.7489, -538.7454) knots 0 0 0 0 0.063398 0.111295 0.111295 0.111295 0.111295
  spline S197 degree 3 poles (26.7489, -538.7454) (26.85, -538.8419) (27.0546, -539.037) (27.3364, -539.0631) (27.4788, -539.0762) knots 0 0 0 0 0.040675 0.082263 0.082263 0.082263 0.082263
  spline S198 degree 3 poles (27.4788, -539.0762) (27.5932, -539.068) (27.816, -539.052) (27.9952, -538.9191) (28.0825, -538.8545) knots 0 0 0 0 0.033628 0.065508 0.065508 0.065508 0.065508
  spline S199 degree 3 poles (28.0825, -538.8545) (28.1565, -538.7645) (28.32, -538.5658) (28.3648, -538.3115) (28.3894, -538.1723) knots 0 0 0 0 0.034396 0.07593 0.07593 0.07593 0.07593
  line L44 (21.9641, -488.1903) -> (22.6087, -488.1357)
  spline S200 degree 3 poles (22.6087, -488.1357) (22.6364, -488.2789) (22.6877, -488.5438) (22.8614, -488.7491) (22.9413, -488.8434) knots 0 0 0 0 0.042908 0.079365 0.079365 0.079365 0.079365
  spline S201 degree 3 poles (22.9413, -488.8434) (23.0334, -488.9125) (23.2201, -489.0525) (23.4528, -489.071) (23.5705, -489.0804) knots 0 0 0 0 0.033826 0.068485 0.068485 0.068485 0.068485
  spline S202 degree 3 poles (23.5705, -489.0804) (23.713, -489.0661) (23.9997, -489.0373) (24.2134, -488.8436) (24.3209, -488.7461) knots 0 0 0 0 0.041772 0.0841 0.0841 0.0841 0.0841
  spline S203 degree 3 poles (24.3209, -488.7461) (24.4103, -488.6211) (24.5995, -488.3566) (24.618, -488.031) (24.6278, -487.8594) knots 0 0 0 0 0.045186 0.095569 0.095569 0.095569 0.095569
  spline S204 degree 3 poles (24.6278, -487.8594) (24.6187, -487.697) (24.6017, -487.3907) (24.4187, -487.1457) (24.3328, -487.0306) knots 0 0 0 0 0.047557 0.089725 0.089725 0.089725 0.089725
  spline S205 degree 3 poles (24.3328, -487.0306) (24.2243, -486.9421) (23.9997, -486.7589) (23.71, -486.7379) (23.5603, -486.7271) knots 0 0 0 0 0.040971 0.08482 0.08482 0.08482 0.08482
  spline S206 degree 3 poles (23.5603, -486.7271) (23.4646, -486.7322) (23.2773, -486.7423) (23.1078, -486.8225) (23.0248, -486.8618) knots 0 0 0 0 0.028423 0.055689 0.055689 0.055689 0.055689
  spline S207 degree 3 poles (23.0248, -486.8618) (22.9499, -486.9093) (22.8031, -487.0026) (22.7001, -487.1427) (22.6496, -487.2114) knots 0 0 0 0 0.026342 0.051681 0.051681 0.051681 0.051681
  line L45 (22.6496, -487.2114) -> (22.0732, -487.1364)
  line L46 (22.0732, -487.1364) -> (22.5575, -484.5681)
  line L47 (22.5575, -484.5681) -> (25.0438, -484.5681)
  line L48 (25.0438, -484.5681) -> (25.0439, -485.1547)
  line L49 (25.0439, -485.1547) -> (23.0486, -485.1548)
  line L50 (23.0486, -485.1548) -> (22.7792, -486.4986)
  spline S208 degree 3 poles (22.7792, -486.4986) (22.9287, -486.4071) (23.2196, -486.229) (23.559, -486.1992) (23.724, -486.1848) knots 0 0 0 0 0.051785 0.100763 0.100763 0.100763 0.100763
  spline S209 degree 3 poles (23.724, -486.1848) (23.9332, -486.2031) (24.3488, -486.2396) (24.6697, -486.5061) (24.829, -486.6384) knots 0 0 0 0 0.061424 0.122014 0.122014 0.122014 0.122014
  spline S210 degree 3 poles (24.829, -486.6384) (24.9603, -486.8038) (25.2311, -487.1451) (25.2629, -487.5805) (25.2792, -487.8048) knots 0 0 0 0 0.061868 0.127641 0.127641 0.127641 0.127641
  spline S211 degree 3 poles (25.2792, -487.8048) (25.264, -488.0217) (25.2342, -488.4476) (24.999, -488.8035) (24.8836, -488.9781) knots 0 0 0 0 0.064036 0.125703 0.125703 0.125703 0.125703
  spline S212 degree 3 poles (24.8836, -488.9781) (24.7059, -489.1551) (24.3428, -489.5168) (23.8315, -489.5621) (23.5705, -489.5852) knots 0 0 0 0 0.072854 0.148822 0.148822 0.148822 0.148822
  spline S213 degree 3 poles (23.5705, -489.5852) (23.3573, -489.5724) (22.9498, -489.5481) (22.6161, -489.3145) (22.4569, -489.2032) knots 0 0 0 0 0.062678 0.119794 0.119794 0.119794 0.119794
  spline S214 degree 3 poles (22.4569, -489.2032) (22.3283, -489.0628) (22.064, -488.7745) (21.998, -488.3884) (21.9641, -488.1903) knots 0 0 0 0 0.055877 0.114795 0.114795 0.114795 0.114795
  line L51 (28.3829, -488.1731) -> (28.9866, -488.2515)
  spline S215 degree 3 poles (28.9866, -488.2515) (28.9439, -488.4455) (28.8622, -488.8172) (28.6037, -489.0955) (28.4801, -489.2287) knots 0 0 0 0 0.058356 0.111856 0.111856 0.111856 0.111856
  spline S216 degree 3 poles (28.4801, -489.2287) (28.3341, -489.3316) (28.034, -489.5431) (27.6673, -489.5686) (27.4791, -489.5817) knots 0 0 0 0 0.052559 0.107965 0.107965 0.107965 0.107965
  spline S217 degree 3 poles (27.4791, -489.5817) (27.2461, -489.5642) (26.7945, -489.5303) (26.4502, -489.2374) (26.2837, -489.0957) knots 0 0 0 0 0.068154 0.132052 0.132052 0.132052 0.132052
  spline S218 degree 3 poles (26.2837, -489.0957) (26.1521, -488.905) (25.8643, -488.4876) (25.8432, -487.9788) (25.8318, -487.7025) knots 0 0 0 0 0.068157 0.149141 0.149141 0.149141 0.149141
  spline S219 degree 3 poles (25.8318, -487.7025) (25.8381, -487.5172) (25.8501, -487.1647) (25.9695, -486.8332) (26.0261, -486.6759) knots 0 0 0 0 0.055211 0.105055 0.105055 0.105055 0.105055
  spline S220 degree 3 poles (26.0261, -486.6759) (26.0983, -486.539) (26.2405, -486.2693) (26.4934, -486.0995) (26.6179, -486.0159) knots 0 0 0 0 0.04564 0.089884 0.089884 0.089884 0.089884
  spline S221 degree 3 poles (26.6179, -486.0159) (26.7538, -485.9517) (27.0277, -485.8224) (27.3301, -485.8048) (27.4825, -485.7959) knots 0 0 0 0 0.044643 0.089955 0.089955 0.089955 0.089955
  spline S222 degree 3 poles (27.4825, -485.7959) (27.6662, -485.8053) (28.0141, -485.823) (28.3087, -486.0073) (28.4477, -486.0943) knots 0 0 0 0 0.054149 0.102527 0.102527 0.102527 0.102527
  spline S223 degree 3 poles (28.4477, -486.0943) (28.5622, -486.2078) (28.8012, -486.4448) (28.885, -486.7716) (28.9286, -486.9418) knots 0 0 0 0 0.047449 0.099081 0.099081 0.099081 0.099081
  line L52 (28.9286, -486.9418) -> (28.3317, -487.0339)
  spline S224 degree 3 poles (28.3317, -487.0339) (28.3009, -486.9226) (28.2434, -486.7151) (28.0975, -486.5577) (28.0299, -486.4848) knots 0 0 0 0 0.034086 0.063475 0.063475 0.063475 0.063475
  spline S225 degree 3 poles (28.0299, -486.4848) (27.9529, -486.4311) (27.7956, -486.3214) (27.6041, -486.3077) (27.5064, -486.3007) knots 0 0 0 0 0.027619 0.056426 0.056426 0.056426 0.056426
  spline S226 degree 3 poles (27.5064, -486.3007) (27.3597, -486.3137) (27.0706, -486.3394) (26.8576, -486.5362) (26.7526, -486.6332) knots 0 0 0 0 0.04285 0.084486 0.084486 0.084486 0.084486
  spline S227 degree 3 poles (26.7526, -486.6332) (26.6684, -486.7728) (26.4745, -487.0943) (26.467, -487.4718) (26.4627, -487.6854) knots 0 0 0 0 0.048123 0.11083 0.11083 0.11083 0.11083
  spline S228 degree 3 poles (26.4627, -487.6854) (26.4663, -487.9012) (26.4726, -488.2799) (26.6612, -488.6058) (26.7424, -488.7461) knots 0 0 0 0 0.063398 0.111295 0.111295 0.111295 0.111295
  spline S229 degree 3 poles (26.7424, -488.7461) (26.8436, -488.8426) (27.0481, -489.0377) (27.3299, -489.0638) (27.4723, -489.0769) knots 0 0 0 0 0.040675 0.082263 0.082263 0.082263 0.082263
  spline S230 degree 3 poles (27.4723, -489.0769) (27.5867, -489.0687) (27.8095, -489.0527) (27.9888, -488.9199) (28.076, -488.8552) knots 0 0 0 0 0.033628 0.065508 0.065508 0.065508 0.065508
  spline S231 degree 3 poles (28.076, -488.8552) (28.15, -488.7652) (28.3135, -488.5666) (28.3584, -488.3122) (28.3829, -488.1731) knots 0 0 0 0 0.034396 0.07593 0.07593 0.07593 0.07593
  spline S232 degree 3 poles (22.0707, -437.0337) (22.0743, -436.7654) (22.0808, -436.2822) (22.2, -435.8144) (22.2531, -435.6064) knots 0 0 0 0 0.080152 0.144341 0.144341 0.144341 0.144341
  spline S233 degree 3 poles (22.2531, -435.6064) (22.3177, -435.4395) (22.4402, -435.123) (22.6813, -434.885) (22.7953, -434.7724) knots 0 0 0 0 0.052977 0.10048 0.10048 0.10048 0.10048
  spline S234 degree 3 poles (22.7953, -434.7724) (22.9267, -434.6869) (23.2015, -434.508) (23.5295, -434.489) (23.7008, -434.479) knots 0 0 0 0 0.046203 0.096661 0.096661 0.096661 0.096661
  spline S235 degree 3 poles (23.7008, -434.479) (23.8286, -434.4846) (24.0741, -434.4953) (24.2989, -434.5938) (24.4068, -434.641) knots 0 0 0 0 0.037989 0.072993 0.072993 0.072993 0.072993
  spline S236 degree 3 poles (24.4068, -434.641) (24.504, -434.7017) (24.7014, -434.8249) (24.8386, -435.0128) (24.9082, -435.1082) knots 0 0 0 0 0.034048 0.069103 0.069103 0.069103 0.069103
  spline S237 degree 3 poles (24.9082, -435.1082) (24.9715, -435.2192) (25.1055, -435.4541) (25.1796, -435.7144) (25.2186, -435.8517) knots 0 0 0 0 0.038176 0.080832 0.080832 0.080832 0.080832
  spline S238 degree 3 poles (25.2186, -435.8517) (25.2513, -436.0228) (25.3259, -436.4129) (25.3294, -436.8103) (25.3313, -437.0335) knots 0 0 0 0 0.052146 0.118926 0.118926 0.118926 0.118926
  spline S239 degree 3 poles (25.3313, -437.0335) (25.3276, -437.3001) (25.3211, -437.7809) (25.2032, -438.2466) (25.1506, -438.454) knots 0 0 0 0 0.079639 0.143634 0.143634 0.143634 0.143634
  spline S240 degree 3 poles (25.1506, -438.454) (25.0864, -438.621) (24.9646, -438.938) (24.724, -439.1767) (24.6101, -439.2897) knots 0 0 0 0 0.052961 0.100531 0.100531 0.100531 0.100531
  spline S241 degree 3 poles (24.6101, -439.2897) (24.4785, -439.3757) (24.2028, -439.5558) (23.8733, -439.5748) (23.7012, -439.5848) knots 0 0 0 0 0.046338 0.097057 0.097057 0.097057 0.097057
  spline S242 degree 3 poles (23.7012, -439.5848) (23.4749, -439.5655) (23.0337, -439.5278) (22.7188, -439.2176) (22.5654, -439.0664) knots 0 0 0 0 0.065835 0.128409 0.128409 0.128409 0.128409
  spline S243 degree 3 poles (22.5654, -439.0664) (22.4219, -438.7984) (22.0843, -438.1674) (22.0757, -437.4477) (22.0707, -437.0337) knots 0 0 0 0 0.090022 0.211899 0.211899 0.211899 0.211899
  line L53 (28.4896, -438.1724) -> (29.0933, -438.2508)